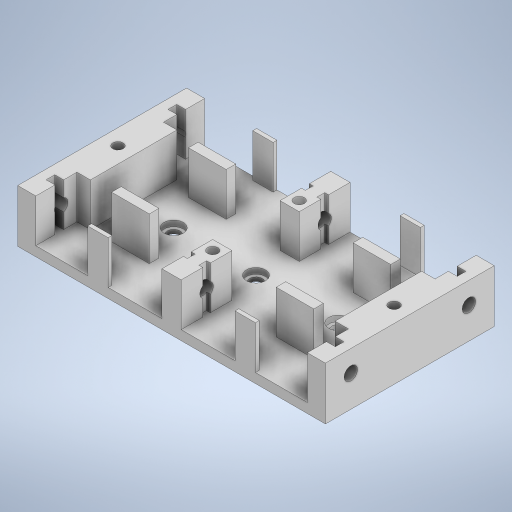
# Autodesk Inventor part: PROJECT SCHOOL
Saved by Autodesk Inventor 2024 (Build 280153000, 153)
## iProperties
Created: 2025-05-09
Part Number: PROJECT SCHOOL
Material: Generic
Document SubType Name: Modeling
Designer: arikm
Density: 1 g/cm^3
Appearance: Default
Author: arikm
Autodesk Inventor part; units mm, degrees
ref_plane "YZ Plane" through (0, 0, 0) normal (1, 0, 0) x (0, 1, 0)
ref_plane "XZ Plane" through (0, 0, 0) normal (0, 1, 0) x (-1, 0, 0)
ref_plane "XY Plane" through (0, 0, 0) normal (0, 0, 1) x (1, 0, 0)
sketch "Sketch1" plane through (0, 0, 0) normal (0, 1, 0) x (-1, 0, 0)
  line L0 (0, 0) -> (-70, 0)
  line L1 (-70, 0) -> (-70, -19.4)
  line L2 (-70, -19.4) -> (0, -19.4)
  line L3 (0, -19.4) -> (0, 0)
  line L4 (0, 0) -> (-4.4, 0)
  line L5 (-4.4, 0) -> (-4.4, -19.4)
  line L6 (-4.4, -19.4) -> (0, -19.4)
  line L7 (0, -19.4) -> (0, 0)
  line L8 (0, -9.7) -> (-4.4, -9.7)
  line L9 (0, -7.95) -> (-4.4, -7.95)
  line L10 (0, -11.45) -> (-4.4, -11.45)
  line L11 (5, -24.4) -> (-75, -24.4)
  line L12 (-75, -24.4) -> (-75, 5)
  line L13 (-75, 5) -> (5, 5)
  line L14 (5, 5) -> (5, -24.4)
  line L15 (-75, 0) -> (-75, 2)
  line L16 (-75, 2) -> (5, 2)
  dimension "d0" = 70
  dimension "d1" = 19.4
  dimension "d2" = 4.4
  dimension "d3" = 1.75
  dimension "d4" = 1.75
  dimension "d5" = 5
  dimension "d6" = 2
  constraints: 34 end point, 8 parallel, 4 perpendicular, 4 point on line, 2 horizontal, 2 midpoint, 3 other
  measures "d0" distance of L2.end L1.end
  measures "d1" distance of L1.end L0.end
  measures "d2" distance of L6.end L5.end
  measures "d3" distance between parallel lines of L8 L9
  measures "d4" distance between parallel lines of L8 L10
  measures "d5" distance between parallel lines of L2 L11
  measures "d6" distance of L15.start L15.end
extrude "Extrusion1" add sketch "Sketch1" along normal blind 22.4 contours L3 L9 L5 L0 | L3 L2 L5 L10 | L11 L12 L16 L14
sketch "Sketch2" plane through (0, 0, 0) normal (0, -1, 0) x (1, 0, 0)
  line L0 (-5, -24.4) -> (-5, 2) projected
  line L1 (75, -24.4) -> (-5, -24.4) projected
  line L2 (-5, 2) -> (75, 2)
  line L3 (75, 2) -> (75, -24.4)
  line L4 (75, -24.4) -> (-5, -24.4)
  line L5 (-5, -24.4) -> (-5, 2)
  point P0 (0, 0)
  constraints: 8 end point, 2 parallel, 1 horizontal, 1 perpendicular
extrude "Extrusion2" add sketch "Sketch2" along normal blind 1
sketch "Sketch3" plane through (0, 22.4, 0) normal (0, 1, 0) x (1, 0, 0)
  line L0 (75, -2) -> (75, 24.4) projected
  line L1 (75, 24.4) -> (48, 24.4)
  line L2 (48, 24.4) -> (48, -5.6)
  line L3 (48, -5.6) -> (75, -5.6)
  line L4 (75, -5.6) -> (75, 24.4)
  point P0 (0, 0)
  dimension "d11" = 27
  dimension "d12" = 30
  constraints: 8 end point, 2 parallel, 1 horizontal, 1 perpendicular
  measures "d11" distance of L3.end L2.end
  measures "d12" distance of L2.end L1.end
extrude "Extrusion3" cut sketch "Sketch3" against normal up to surface (22.4 mm away)
sketch "Sketch4" plane through (0, 22.4, 0) normal (0, 1, 0) x (1, 0, 0)
  line L0 (48, 0) -> (4.4, 0) projected
  line L1 (4.4, 0) -> (13.4, 0)
  line L2 (13.4, 0) -> (12.4, 0)
  line L3 (12.4, 0) -> (17.4, 0)
  line L4 (17.4, 0) -> (12.4, 0)
  line L5 (12.4, 0) -> (12.4, -8.176)
  line L6 (12.4, -8.176) -> (17.4, -8.176)
  line L7 (17.4, -8.176) -> (17.4, 0)
  line L8 (12.4, -8.176) -> (17.4, -8.176)
  line L9 (17.4, -8.176) -> (17.4, 29.1171)
  line L10 (17.4, 29.1171) -> (12.4, 29.1171)
  line L11 (12.4, 29.1171) -> (12.4, -8.176)
  point P0 (0, 0)
  dimension "d15" = 9
  dimension "d16" = 1
  dimension "d17" = 5
  constraints: 22 end point, 4 parallel, 4 point on line, 2 horizontal, 2 perpendicular
  measures "d15" distance of L0.end L1.end
  measures "d16" distance of L1.end L2.end
  measures "d17" distance of L2.end L3.end
extrude "Extrusion4" cut sketch "Sketch4" against normal up to surface (22.4 mm away)
sketch "Sketch5" plane through (-5, -1, 2) normal (0, 0, 1) x (1, 0, 0)
  line L0 (17.4, 1) -> (22.4, 1) projected
  line L1 (53, 23.4) -> (22.4, 23.4) projected
  line L2 (17.4, 1) -> (27.4, 1)
  line L3 (27.4, 1) -> (27.4, 23.4)
  line L4 (27.4, 23.4) -> (17.4, 23.4)
  line L5 (17.4, 23.4) -> (17.4, 1)
  point P0 (5, 1)
  dimension "d20" = 10
  constraints: 8 end point, 2 parallel, 1 horizontal, 1 perpendicular, 1 point on line
  measures "d20" distance of L4.end L3.end
extrude "Extrusion5" cut sketch "Sketch5" against normal through all
sketch "Sketch6" plane through (-5, -1, 2) normal (0, 0, 1) x (1, 0, 0)
  line L0 (17.4, 23.4) -> (17.4, 1) projected
  line L1 (17.4, 23.4) -> (9.4, 23.4)
  line L2 (17.4, 23.4) -> (0, 23.4) projected
  line L3 (53, 23.4) -> (27.4, 23.4) projected
  line L4 (27.4, 23.4) -> (35.4, 23.4)
  line L5 (9.4, 23.4) -> (35.4, 23.4)
  line L6 (35.4, 23.4) -> (35.4, 1)
  line L7 (35.4, 1) -> (9.4, 1)
  line L8 (9.4, 1) -> (9.4, 23.4)
  point P0 (5, 1)
  dimension "d23" = 8
  dimension "d24" = 8
  constraints: 12 end point, 2 parallel, 2 point on line, 1 horizontal, 1 perpendicular
  measures "d23" distance of L0.start L1.end
  measures "d24" distance of L3.end L4.end
extrude "Extrusion6" cut sketch "Sketch6" against normal blind 10
sketch "Sketch7" plane through (0, 0, 0) normal (0, 1, 0) x (1, 0, 0)
  line L0 (-5, 24.4) -> (75, 24.4) projected
  line L1 (75, 24.4) -> (75, 59.4)
  line L2 (75, -2) -> (-5, -2) projected
  line L3 (75, -2) -> (-5, -2)
  line L4 (-5, -2) -> (-5, 24.4)
  line L5 (-5, 24.4) -> (75, 24.4)
  line L6 (75, 24.4) -> (75, -2)
  line L7 (4.4, -2) -> (4.4, 7.95) projected
  line L8 (4.4, 7.95) -> (4.4, -2)
  line L9 (4.4, 7.95) -> (0, 7.95)
  line L10 (0, 7.95) -> (0, 11.45) projected
  line L11 (0, 7.95) -> (0, 11.45)
  line L12 (0, 11.45) -> (4.4, 11.45)
  line L13 (4.4, 11.45) -> (4.4, 19.4) projected
  line L14 (0, 11.45) -> (4.4, 11.45)
  line L15 (4.4, 11.45) -> (4.4, 19.4)
  line L16 (12.4, 19.4) -> (12.4, 24.4) projected
  line L17 (4.4, 19.4) -> (12.4, 19.4)
  line L18 (12.4, 19.4) -> (12.4, 24.4)
  line L19 (22.4, 19.4) -> (22.4, 24.4) projected
  line L20 (12.4, 24.4) -> (22.4, 24.4)
  line L21 (22.4, 19.4) -> (48, 19.4) projected
  line L22 (22.4, 24.4) -> (48, 24.4)
  line L23 (48, 24.4) -> (48, 19.4)
  line L24 (48, 19.4) -> (22.4, 19.4)
  line L25 (22.4, 19.4) -> (22.4, 24.4)
  line L26 (75, 41.9) -> (-5, 41.9)
  line L27 (48, 0) -> (30.4, 0) projected
  line L28 (30.4, -2) -> (48, -2)
  line L29 (48, -2) -> (48, 0)
  line L30 (48, 0) -> (30.4, 0)
  line L31 (30.4, 0) -> (30.4, -2)
  line L32 (-5, 59.4) -> (75, 59.4)
  line L33 (75, 85.8) -> (-5, 85.8)
  line L34 (-5, 85.8) -> (-5, 59.4)
  line L35 (75, 59.4) -> (75, 85.8)
  line L36 (4.4, 75.85) -> (4.4, 85.8)
  line L37 (4.4, 75.85) -> (0, 75.85)
  line L38 (0, 75.85) -> (0, 72.35)
  line L39 (0, 72.35) -> (4.4, 72.35)
  line L40 (4.4, 72.35) -> (4.4, 64.4)
  line L41 (12.4, 64.4) -> (12.4, 59.4)
  line L42 (4.4, 64.4) -> (12.4, 64.4)
  line L43 (22.4, 64.4) -> (22.4, 59.4)
  line L44 (48, 59.4) -> (48, 64.4)
  line L45 (48, 64.4) -> (22.4, 64.4)
  line L46 (48, 83.8) -> (30.4, 83.8)
  line L47 (48, 85.8) -> (48, 83.8)
  line L48 (30.4, 83.8) -> (30.4, 85.8)
  point P0 (0, 0)
  dimension "d27" = 35
  constraints: 80 end point, 24 symmetric about line, 7 perpendicular, 6 parallel, 5 horizontal, 4 collinear, 1 midpoint, 1 point on line, 1 vertical
  measures "d27" distance of L0.end L1.end
extrude "Extrusion7" add sketch "Sketch7" against normal blind 1 contours L34 L33 L36 L37 L38 L39 L40 L42 L41 L32 | L41 L42 L40 L39 L38 L37 L36 L33 L48 L46 L47 L35 L32 L44 L45 L43 | L43 L45 L44 L32 | L33 L47 L46 L48
extrude "Extrusion8" add sketch "Sketch7" along normal up to surface (22.4 mm away) contours L34 L33 L36 L37 L38 L39 L40 L42 L41 L32 | L43 L45 L44 L32 | L33 L47 L46 L48
thicken "Thicken1" operation cut thickness 1 both sides no extend neighbours no toward (1, 0, 0) faces at (30.4, 7.4667, 0.6667)
thicken "Thicken2" operation cut thickness 1 both sides no extend neighbours no toward (1, 0, 0) faces at (30.4, 7.4667, -85.1333)
thicken "Thicken3" operation cut thickness 1 both sides no extend neighbours no toward (-1, 0, 0) faces at (12.4, 7.4667, -22.7333)
thicken "Thicken4" operation cut thickness 1 both sides no extend neighbours no toward (-1, 0, 0) faces at (12.4, 7.4667, -61.0667)
thicken "Thicken7" operation cut thickness 0.2 both sides no extend neighbours no toward (-1, 0, 0) faces at (0, 7.4667, -9.1167)
thicken "Thicken8" operation cut thickness 0.2 both sides no extend neighbours no toward (-1, 0, 0) faces at (0, 7.4667, -73.5167)
sketch "Sketch8" plane through (0, 22.4, 0) normal (0, 1, 0) x (1, 0, 0)
  line L0 (48, 0) -> (48, -2) projected
  line L1 (-5, 85.8) -> (75, 85.8) projected
  line L2 (48, -2) -> (42, -2)
  line L3 (42, -2) -> (42, 85.8)
  line L4 (42, 85.8) -> (48, 85.8)
  line L5 (48, 85.8) -> (48, -2)
  point P0 (0, 0)
  dimension "d48" = 6
  constraints: 8 end point, 2 parallel, 1 horizontal, 1 perpendicular, 1 point on line
  measures "d48" distance of L3.end L4.end
extrude "Extrusion9" cut sketch "Sketch8" against normal up to surface (22.4 mm away)
sketch "Sketch9" plane through (0, 0, 0) normal (0, 1, 0) x (1, 0, 0)
  line L0 (75, 24.4) -> (75, -2) projected
  line L1 (-5, 24.4) -> (75, 24.4) projected
  line L2 (75, -2) -> (70, -2)
  line L3 (70, -2) -> (70, 24.4)
  line L4 (70, 24.4) -> (75, 24.4)
  line L5 (75, 24.4) -> (75, -2)
  line L6 (75, 59.4) -> (75, 85.8) projected
  line L7 (-5, 85.8) -> (75, 85.8) projected
  line L8 (75, 59.4) -> (70, 59.4)
  line L9 (70, 59.4) -> (70, 85.8)
  line L10 (70, 85.8) -> (75, 85.8)
  line L11 (75, 85.8) -> (75, 59.4)
  point P0 (0, 0)
  dimension "d51" = 5
  dimension "d52" = 5
  constraints: 16 end point, 4 parallel, 2 horizontal, 2 perpendicular, 2 point on line
  measures "d51" distance of L3.end L4.end
  measures "d52" distance of L9.end L10.end
extrude "Extrusion10" add sketch "Sketch9" along normal up to surface (22.4 mm away)
sketch "Sketch10" plane through (75, -1, 2) normal (1, 0, 0) x (0, 0, -1)
  line L0 (2, 1) -> (0, 1) projected
  line L1 (26.4, 23.4) -> (26.4, 1) projected
  line L2 (0, 1) -> (26.4, 1)
  line L3 (26.4, 1) -> (26.4, 23.4)
  line L4 (26.4, 23.4) -> (0, 23.4)
  line L5 (0, 23.4) -> (0, 1)
  line L6 (0, 12.2) -> (87.8, 12.2)
  line L7 (87.8, 1) -> (87.8, 23.4) projected
  line L8 (61.4, 0) -> (61.4, 23.4) projected
  line L9 (61.4, 12.2) -> (87.8, 12.2)
  circle A0 centre (13.2, 12.2) radius 3.5
  circle A1 centre (74.6, 12.2) radius 3.5
  dimension "d55" = 7
  dimension "d56" = 7
  constraints: 12 end point, 3 midpoint, 3 point on line, 2 centre point, 2 parallel, 1 collinear, 1 horizontal, 1 perpendicular
  measures "d55" diameter of A0
  measures "d56" diameter of A1
extrude "Extrusion11" cut sketch "Sketch10" against normal through all contours A0 L6 | L6 A0 | A1 L6 | L6 A1
sketch "Sketch11" plane through (70, 22.4, 2) normal (0, 1, 0) x (1, 0, 0)
  line L0 (0, 0) -> (0, 26.4) projected
  line L1 (0, 13.2) -> (2, 13.2)
  line L2 (0, 13.2) -> (2, 13.2) construction
  line L3 (2, 13.2) -> (0, 13.2)
  line L4 (0, 13.2) -> (0, 11.2)
  line L5 (0, 11.2) -> (2, 11.2)
  line L6 (2, 11.2) -> (2, 13.2)
  line L7 (0, 11.2) -> (2, 11.2)
  line L8 (2, 11.2) -> (2, 15.2)
  line L9 (2, 15.2) -> (0, 15.2)
  line L10 (0, 15.2) -> (0, 11.2)
  line L11 (0, 61.4) -> (0, 87.8) projected
  line L12 (0, 74.6) -> (2, 74.6)
  line L13 (2, 74.6) -> (2, 73.4639)
  line L14 (2, 73.4639) -> (0, 73.4639)
  line L15 (0, 73.4639) -> (0, 74.6)
  line L16 (2, 74.6) -> (0, 74.6)
  line L17 (0, 74.6) -> (0, 76.6)
  line L18 (0, 76.6) -> (2, 76.6)
  line L19 (2, 76.6) -> (2, 74.6)
  line L20 (0, 74.6) -> (2, 74.6)
  line L21 (2, 74.6) -> (2, 72.6)
  line L22 (2, 72.6) -> (0, 72.6)
  line L23 (0, 72.6) -> (0, 74.6)
  point P0 (-70, 2)
  point P1 (2, 13.2)
  point P2 (0, 15.2)
  point P3 (2, 73.4639)
  dimension "d59" = 2
  dimension "d60" = 0
  dimension "d61" = 2
  dimension "d62" = 4
  dimension "d63" = 2
  dimension "d64" = 2
  dimension "d65" = 2
  constraints: 44 end point, 10 parallel, 7 horizontal, 5 perpendicular, 4 point on line, 2 midpoint, 1 collinear
  measures "d59" distance of L1.start L1.end
  measures "d60" distance between parallel lines of L1 L2
  measures "d61" distance of L4.end L3.end
  measures "d62" distance of L8.end L7.end
  measures "d63" distance of L13.end L14.end
  measures "d64" distance of L16.end L17.end
  measures "d65" distance of L20.end L21.end
extrude "Extrusion12" cut sketch "Sketch11" against normal up to surface contours L0 L1 L6 L5 | L0 L9 L8 L1 round surface about axis through (75, 11.2, -11.2) along (-1, 0, 0) radius 3.5 far side no
extrude "Extrusion13" cut sketch "Sketch11" against normal up to surface contours L11 L14 L21 L22 | L11 L12 L13 L14 | L11 L18 L19 L12 round surface about axis through (75, 11.2, -72.6) along (-1, 0, 0) radius 3.5 far side no
sketch "Sketch12" plane through (0, 22.4, 0) normal (0, 1, 0) x (1, 0, 0)
  line L0 (4.4, 14.7) -> (4.4, 11.45) projected
  line L1 (-0.2, 11.45) -> (4.4, 11.45)
  line L2 (4.4, 11.45) -> (4.4, 12.45)
  line L3 (4.4, 12.45) -> (-0.2, 12.45)
  line L4 (-0.2, 12.45) -> (-0.2, 11.45)
  point P0 (0, 0)
  dimension "d70" = 1
  constraints: 8 end point, 2 parallel, 1 horizontal, 1 perpendicular, 1 point on line
  measures "d70" distance of L2.end L1.end
extrude "Extrusion14" cut sketch "Sketch12" against normal up to surface (22.4 mm away)
sketch "Sketch13" plane through (-5, 22.4, -85.8) normal (0, 1, 0) x (1, 0, 0)
  line L0 (9.4, -13.45) -> (9.4, -21.4) projected
  line L1 (9.4, -13.45) -> (4.8, -13.45)
  line L2 (4.8, -13.45) -> (4.8, -14.45)
  line L3 (4.8, -14.45) -> (9.4, -14.45)
  line L4 (9.4, -14.45) -> (9.4, -13.45)
  point P0 (5, -85.8)
  point P1 (9.4, -14.45)
  dimension "d73" = 1
  constraints: 8 end point, 2 parallel, 1 horizontal, 1 perpendicular
  measures "d73" distance of L2.end L1.end
extrude "Extrusion15" cut sketch "Sketch13" against normal up to surface (22.4 mm away)
sketch "Sketch14" plane through (0, 0, 0) normal (0, 1, 0) x (1, 0, 0)
  line L0 (11.4, 24.4) -> (-5, 24.4) projected
  line L1 (75, 59.4) -> (-5, 59.4) projected
  line L2 (-5, 24.4) -> (75, 24.4)
  line L3 (75, 24.4) -> (75, 59.4)
  line L4 (75, 59.4) -> (-5, 59.4)
  line L5 (-5, 59.4) -> (-5, 24.4)
  point P0 (0, 0)
  constraints: 8 end point, 2 parallel, 1 horizontal, 1 perpendicular
extrude "Extrusion16" add sketch "Sketch14" against normal up to surface (1 mm away)
sketch "Sketch15" plane through (0, 0, 0) normal (0, 1, 0) x (1, 0, 0)
  line L0 (-5, -2) -> (-5, 85.8) projected
  line L1 (75, 85.8) -> (75, -2) projected
  line L2 (-5, -2) -> (75, -2)
  line L3 (75, -2) -> (75, 85.8)
  line L4 (75, 85.8) -> (-5, 85.8)
  line L5 (-5, 85.8) -> (-5, -2)
  line L6 (-0.2, 7.95) -> (-0.2, 12.45) projected
  line L7 (-0.2, 12.45) -> (4.4, 12.45) projected
  line L8 (-0.2, 7.95) -> (4.4, 7.95)
  line L9 (4.4, 7.95) -> (4.4, 12.45)
  line L10 (4.4, 12.45) -> (-0.2, 12.45)
  line L11 (-0.2, 12.45) -> (-0.2, 7.95)
  line L12 (11.4, 24.4) -> (-5, 24.4) projected
  line L13 (4.4, 19.4) -> (11.4, 19.4) projected
  line L14 (-5, 24.4) -> (11.4, 24.4)
  line L15 (11.4, 24.4) -> (11.4, 19.4)
  line L16 (11.4, 19.4) -> (-5, 19.4)
  line L17 (-5, 19.4) -> (-5, 24.4)
  line L18 (-5, -2) -> (4.4, -2)
  line L19 (4.4, -2) -> (4.4, 19.4)
  line L20 (4.4, 19.4) -> (-5, 19.4)
  line L21 (-5, 19.4) -> (-5, -2)
  line L22 (11.4, 19.4) -> (-5, 19.4)
  line L23 (-5, 19.4) -> (-5, 24.4)
  line L24 (-5, 24.4) -> (11.4, 24.4)
  line L25 (11.4, 24.4) -> (11.4, 19.4)
  line L26 (31.4, -2) -> (31.4, 0) projected
  line L27 (42, 0) -> (31.4, 0) projected
  line L28 (31.4, -2) -> (42, -2)
  line L29 (42, -2) -> (42, 0)
  line L30 (42, 0) -> (31.4, 0)
  line L31 (31.4, 0) -> (31.4, -2)
  line L32 (22.4, 24.4) -> (22.4, 19.4) projected
  line L33 (22.4, 19.4) -> (42, 19.4)
  line L34 (42, 19.4) -> (42, 24.4)
  line L35 (42, 24.4) -> (22.4, 24.4)
  line L36 (22.4, 24.4) -> (22.4, 19.4)
  line L37 (70, 13.2) -> (70, 24.4) projected
  line L38 (75, -2) -> (70, -2)
  line L39 (70, -2) -> (70, 24.4)
  line L40 (70, 24.4) -> (75, 24.4)
  line L41 (75, 24.4) -> (75, -2)
  line L42 (70, 9.2) -> (72, 9.2) projected
  line L43 (72, 13.2) -> (70, 13.2) projected
  line L44 (70, 9.2) -> (72, 9.2)
  line L45 (72, 9.2) -> (72, 13.2)
  line L46 (72, 13.2) -> (70, 13.2)
  line L47 (70, 13.2) -> (70, 9.2)
  line L48 (-5, 59.4) -> (-5, 24.4) projected
  line L49 (-5, 41.9) -> (75, 41.9)
  line L50 (-5, 85.8) -> (-5, -2)
  line L51 (75, -2) -> (75, 85.8)
  line L52 (-5, 85.8) -> (75, 85.8)
  line L53 (-0.2, 75.85) -> (-0.2, 71.35)
  line L54 (-0.2, 71.35) -> (4.4, 71.35)
  line L55 (-0.2, 75.85) -> (4.4, 75.85)
  line L56 (4.4, 75.85) -> (4.4, 71.35)
  line L57 (4.4, 64.4) -> (11.4, 64.4)
  line L58 (-5, 59.4) -> (11.4, 59.4)
  line L59 (4.4, 85.8) -> (4.4, 64.4)
  line L60 (11.4, 59.4) -> (11.4, 64.4)
  line L61 (31.4, 85.8) -> (31.4, 83.8)
  line L62 (42, 83.8) -> (31.4, 83.8)
  line L63 (42, 85.8) -> (42, 83.8)
  line L64 (70, 85.8) -> (70, 59.4)
  line L65 (70, 59.4) -> (75, 59.4)
  line L66 (70, 74.6) -> (72, 74.6)
  line L67 (72, 70.6) -> (70, 70.6)
  line L68 (72, 74.6) -> (72, 70.6)
  line L69 (155, -2) -> (155, 85.8)
  line L70 (155, -2) -> (75, -2)
  line L71 (75, 85.8) -> (155, 85.8)
  line L72 (150.2, 7.95) -> (150.2, 12.45)
  line L73 (150.2, 12.45) -> (145.6, 12.45)
  line L74 (150.2, 7.95) -> (145.6, 7.95)
  line L75 (138.6, 24.4) -> (155, 24.4)
  line L76 (145.6, 19.4) -> (138.6, 19.4)
  line L77 (138.6, 24.4) -> (138.6, 19.4)
  line L78 (145.6, -2) -> (145.6, 19.4)
  line L79 (155, 19.4) -> (155, -2)
  line L80 (118.6, -2) -> (118.6, 0)
  line L81 (108, -2) -> (108, 0)
  line L82 (108, 0) -> (118.6, 0)
  line L83 (127.6, 24.4) -> (127.6, 19.4)
  line L84 (127.6, 19.4) -> (108, 19.4)
  line L85 (108, 19.4) -> (108, 24.4)
  line L86 (108, 24.4) -> (127.6, 24.4)
  line L87 (80, -2) -> (80, 24.4)
  line L88 (80, 24.4) -> (75, 24.4)
  line L89 (80, 9.2) -> (78, 9.2)
  line L90 (78, 13.2) -> (80, 13.2)
  line L91 (78, 9.2) -> (78, 13.2)
  line L92 (150.2, 75.85) -> (145.6, 75.85)
  line L93 (150.2, 75.85) -> (150.2, 71.35)
  line L94 (150.2, 71.35) -> (145.6, 71.35)
  line L95 (145.6, 75.85) -> (145.6, 71.35)
  line L96 (145.6, 85.8) -> (145.6, 64.4)
  line L97 (155, 59.4) -> (138.6, 59.4)
  line L98 (138.6, 59.4) -> (138.6, 64.4)
  line L99 (145.6, 64.4) -> (138.6, 64.4)
  line L100 (108, 83.8) -> (118.6, 83.8)
  line L101 (108, 85.8) -> (108, 83.8)
  line L102 (118.6, 85.8) -> (118.6, 83.8)
  line L103 (80, 85.8) -> (80, 59.4)
  line L104 (80, 59.4) -> (75, 59.4)
  line L105 (78, 74.6) -> (78, 70.6)
  line L106 (80, 74.6) -> (78, 74.6)
  line L107 (78, 70.6) -> (80, 70.6)
  line L108 (155, 41.9) -> (75, 41.9)
  line L109 (127.6, 19.4) -> (108, 19.4)
  line L110 (108, 19.4) -> (108, 24.4)
  line L111 (108, 24.4) -> (127.6, 24.4)
  line L112 (127.6, 24.4) -> (127.6, 19.4)
  line L113 (127.6, 19.4) -> (108, 19.4)
  line L114 (108, 19.4) -> (108, 24.4)
  line L115 (108, 24.4) -> (127.6, 24.4)
  line L116 (127.6, 24.4) -> (127.6, 19.4)
  line L117 (108, 64.4) -> (108, 59.4)
  line L118 (127.6, 64.4) -> (108, 64.4)
  line L119 (127.6, 59.4) -> (127.6, 64.4)
  line L120 (108, 59.4) -> (127.6, 59.4)
  point P0 (0, 0)
  point P1 (75, -2)
  constraints: 216 end point, 86 symmetric about line, 22 parallel, 12 horizontal, 11 perpendicular, 4 point on line, 3 midpoint
extrude "Extrusion17" add sketch "Sketch15" against normal blind 1 contours L108 L69 L75 L77 L76 L78 L70 L80 L82 L81 L87 L88 L1 | L1 L104 L103 L71 L101 L100 L102 L96 L95 L99 L98 L97 L69 L108 | L1 L71 L103 L106 L105 L107 L104 | L88 L87 L90 L91 L89 L70 L1 | L69 L70 L78 L74 L72 L73 L76 L77 L75 | L97 L98 L99 L96 L94 L93 L92 L71 L69 | L107 L105 L106 L103 | L87 L89 L91 L90 | L81 L82 L80 L70 | L71 L102 L100 L101 | L92 L93 L94 L95 | L78 L73 L72 L74 | L83 L84 L85 L86 | L118 L119 L120 L117
extrude "Extrusion18" add sketch "Sketch15" along normal up to surface (22.4 mm away) contours L1 L71 L103 L106 L105 L107 L104 | L88 L87 L90 L91 L89 L70 L1 | L69 L70 L78 L74 L72 L73 L76 L77 L75 | L97 L98 L99 L96 L94 L93 L92 L71 L69 | L81 L82 L80 L70 | L71 L102 L100 L101 | L83 L84 L85 L86 | L118 L119 L120 L117
sketch "Sketch16" plane through (-5, 22.4, -24.4) normal (-1, 0, 0) x (0, 0, 1)
  arc A0 (-51.45, -9.901) -> (-51.45, -12.499) centre (-48.2, -11.2) ccw projected
  circle A1 centre (-48.2, -11.2) radius 3.5
  circle A2 centre (13.2, -11.2) radius 3.5 projected
  circle A3 centre (13.2, -11.2) radius 3.5
  point P0 (24.4, -22.4)
  constraints: 2 centre point, 2 coincident
extrude "Extrusion19" add sketch "Sketch16" against normal through all
extrude "Extrusion20" cut sketch "Sketch16" against normal through all
sketch "Sketch17" plane through (0, -1, 0) normal (0, -1, 0) x (1, 0, 0)
  line L0 (-5, -85.8) -> (155, -85.8) projected
  line L1 (155, 2) -> (-5, 2)
  line L2 (-5, 2) -> (-5, -85.8)
  line L3 (-5, -85.8) -> (155, -85.8)
  line L4 (155, -85.8) -> (155, 2)
  point P0 (0, 0)
  constraints: 8 end point, 2 parallel, 1 horizontal, 1 perpendicular
extrude "Extrusion21" add sketch "Sketch17" along normal blind 4
sketch "Sketch18" plane through (0, 0, 0) normal (0, 1, 0) x (1, 0, 0)
  line L0 (22.4, 59.4) -> (42, 59.4) projected
  line L1 (32.2, 59.4) -> (32.2, 24.4)
  line L2 (42, 24.4) -> (22.4, 24.4) projected
  line L3 (108, 24.4) -> (127.6, 24.4) projected
  line L4 (117.8, 24.4) -> (117.8, 59.4)
  line L5 (127.6, 59.4) -> (108, 59.4) projected
  line L6 (80, 24.4) -> (70, 24.4) projected
  line L7 (75, 24.4) -> (75, 59.4)
  line L8 (80, 59.4) -> (70, 59.4) projected
  circle A0 centre (32.2, 41.9) radius 3.25
  circle A1 centre (75, 41.9) radius 3.25
  circle A2 centre (117.8, 41.9) radius 3.25
  point P0 (0, 0)
  dimension "d88" = 6.5
  dimension "d89" = 6.5
  dimension "d90" = 6.5
  constraints: 9 midpoint, 6 end point, 3 centre point
  measures "d88" diameter of A0
  measures "d89" diameter of A1
  measures "d90" diameter of A2
extrude "Extrusion22" cut sketch "Sketch18" against normal through all
sketch "Sketch19" plane through (0, 0, 0) normal (0, 1, 0) x (1, 0, 0)
  circle A0 centre (32.2, 41.9) radius 3.25 projected
  circle A1 centre (32.2, 41.9) radius 5
  circle A2 centre (75, 41.9) radius 3.25 projected
  circle A3 centre (75, 41.9) radius 5
  circle A4 centre (117.8, 41.9) radius 3.25 projected
  circle A5 centre (117.8, 41.9) radius 5
  point P0 (0, 0)
  dimension "d93" = 10
  dimension "d94" = 10
  dimension "d95" = 10
  constraints: 3 centre point, 3 coincident
  measures "d93" diameter of A1
  measures "d94" diameter of A3
  measures "d95" diameter of A5
extrude "Extrusion23" cut sketch "Sketch19" against normal blind 3 contours A0 | A1 | A2 | A3 | A4 | A5
sketch "Sketch20" plane through (0, 0, 0) normal (0, 1, 0) x (1, 0, 0)
  circle A0 centre (75, 41.9) radius 5 projected
  circle A1 centre (75, 41.9) radius 100
  line L0 (138.6, 24.4) -> (155, 24.4) projected
  line L1 (146.8, 24.4) -> (146.8, 59.4)
  line L2 (155, 59.4) -> (138.6, 59.4) projected
  line L3 (155, 59.4) -> (138.6, 59.4)
  line L4 (138.6, 59.4) -> (138.6, 24.4)
  line L5 (138.6, 24.4) -> (155, 24.4)
  line L6 (155, 24.4) -> (155, 59.4)
  line L7 (-5, -2) -> (-5, 85.8) projected
  line L8 (11.4, 64.4) -> (11.4, 59.4) projected
  line L9 (-5, 24.4) -> (11.4, 24.4)
  line L10 (11.4, 24.4) -> (11.4, 59.4)
  line L11 (11.4, 59.4) -> (-5, 59.4)
  line L12 (-5, 59.4) -> (-5, 24.4)
  point P0 (0, 0)
  constraints: 18 end point, 4 parallel, 2 horizontal, 2 midpoint, 2 perpendicular, 1 centre point, 1 coincident, 1 point on line
extrude "Extrusion24" add sketch "Sketch20" along normal up to surface (22.4 mm away) contours L4 L2 L1 L0 | L1 L2 L6 L0 | L7 L11 L10 L9
sketch "Sketch21" plane through (0, 22.4, 0) normal (0, 1, 0) x (1, 0, 0)
  line L0 (11.4, 19.4) -> (11.4, 64.4) projected
  line L1 (11.4, 41.9) -> (-5, 41.9)
  line L2 (-5, -2) -> (-5, 85.8) projected
  line L3 (155, 85.8) -> (155, -2) projected
  line L4 (155, 41.9) -> (138.6, 41.9)
  line L5 (138.6, 19.4) -> (138.6, 64.4) projected
  circle A0 centre (3.2, 41.9) radius 2.7
  circle A1 centre (146.8, 41.9) radius 2.7
  line L6 (72, 13.2) -> (70, 13.2) projected
  line L7 (80, 24.4) -> (70, 24.4) projected
  line L8 (70, 13.2) -> (80, 13.2)
  line L9 (80, 13.2) -> (80, 24.4)
  line L10 (80, 24.4) -> (70, 24.4)
  line L11 (70, 24.4) -> (70, 13.2)
  line L12 (75, 24.4) -> (75, 19.4)
  line L13 (80, 59.4) -> (70, 59.4) projected
  line L14 (75, 59.4) -> (75, 64.4)
  circle A2 centre (75, 19.4) radius 2.7
  circle A3 centre (75, 64.4) radius 2.7
  point P0 (0, 0)
  dimension "d101" = 5.4
  dimension "d102" = 5.4
  dimension "d103" = 5
  dimension "d104" = 5
  dimension "d105" = 5.4
  dimension "d106" = 5.4
  constraints: 16 end point, 8 midpoint, 4 centre point, 2 coincident, 2 parallel, 2 vertical, 1 horizontal, 1 perpendicular
  measures "d101" diameter of A0
  measures "d102" diameter of A1
  measures "d103" distance of L12.start L12.end
  measures "d104" distance of L14.start L14.end
  measures "d105" diameter of A2
  measures "d106" diameter of A3
extrude "Extrusion25" cut sketch "Sketch21" against normal blind 6 contours A0 L1 | L1 A0 | A1 L4 | L4 A1 | A2 | A3
body "Solid1"
